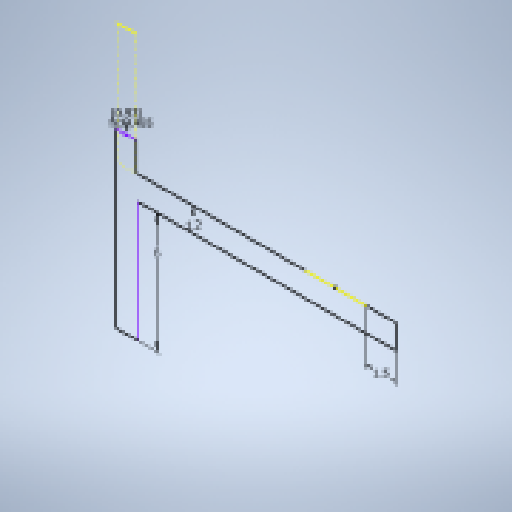
# Autodesk Inventor part: j1 endstop blocker
Saved by Autodesk Inventor 2025 (Build 290162000, 162)
## iProperties
Created: 2025-07-05
Part Number: j1 endstop blocker
Material: 一般
Document SubType Name: Modeling
Designer: gavin
Density: 1 g/cm^3
Appearance: 預設
Author: gavin
Autodesk Inventor part; units mm, degrees
ref_plane "YZ Plane" through (0, 0, 0) normal (1, 0, 0) x (0, 1, 0)
ref_plane "XZ Plane" through (0, 0, 0) normal (0, 1, 0) x (-1, 0, 0)
ref_plane "XY Plane" through (0, 0, 0) normal (0, 0, 1) x (1, 0, 0)
sketch "草圖1" plane through (0, 0, 0) normal (0, 0, 1) x (1, 0, 0)
  line L0 (0, 6) -> (-0.93, 6) projected
  line L1 (0, 0) -> (0, 6) construction
  line L2 (-0.93, 0) -> (0, 0) construction
  line L3 (-0.93, 0) -> (-0.93, 6) construction
  line L4 (-0.965, -0.0008) -> (-0.965, -7.2)
  line L5 (-0.965, -7.2) -> (0.129, -7.2)
  line L6 (0.129, -7.2) -> (0.129, -1.2)
  line L7 (11.5, 0) -> (8.5, 0) projected
  line L8 (0.129, -1.2) -> (13, -1.2)
  line L9 (13, -1.2) -> (13, 0)
  line L10 (13, 0) -> (0.035, 0)
  line L11 (0.035, 0) -> (0.035, 3)
  line L12 (0.035, 3) -> (-0.965, 3)
  line L13 (-0.965, 3) -> (-0.965, -0.0008)
  point P0 (-0.465, 3)
  point P1 (10, 0)
  dimension "d0" = 1
  dimension "d1" = 0.465
  dimension "d2" = 0.93
  dimension "d3" = 1.2
  dimension "d5" = 6
  dimension "d6" = 1.5
  dimension "d7" = 3
  constraints: 18 end point, 6 perpendicular, 2 midpoint, 1 collinear, 1 horizontal, 1 point on line, 1 vertical
  measures "d0" distance of L11.end L12.end
  measures "d1" distance from line of L1 point (-0.465, 3)
  measures "d2" distance between parallel lines of L1 L3
  measures "d3" distance between parallel lines of L8 L10
  measures "d5" distance of L5.end L6.end
  measures "d6" distance from line of L7.start L9
  measures "d7" distance of L10.end L11.end
extrude "擠出1" add sketch "草圖1" along normal blind 6
sketch "草圖2" plane through (0.129, -1.2, 0) normal (0, -1, 0) x (1, 0, 0)
  circle A0 centre (9.871, 3) radius 1.5 projected
  point P0 (-0.129, 0)
extrude "擠出2" cut sketch "草圖2" against normal blind 4.2
fillet "圓角1" radius 3 2 edges at (13, -0.6, 6) (13, -0.6, 0)
equation "\"d1\" = 0.5 * d2"
